Autodesk Fusion 360 part; units mm, degrees
(part 3 of 3)
sketch "Sketch9" plane through (0, 0, 0) normal (1, 0, 0) x (0, 1, 0)
  line L0 (143.1111, 10) -> (156, 10)
  line L1 (156, 10) -> (156, 27)
  line L2 (156, 27) -> (161, 27)
  line L3 (161, 27) -> (161, 49)
  line L4 (161, 49) -> (156, 49)
  line L5 (156, 49) -> (156, 71)
  line L6 (156, 71) -> (161, 71)
  line L7 (161, 71) -> (161, 93)
  line L8 (161, 93) -> (156, 93)
  line L9 (156, 93) -> (156, 115)
  line L10 (156, 115) -> (5, 115)
  line L11 (5, 115) -> (5, 93)
  line L12 (5, 93) -> (0, 93)
  line L13 (0, 93) -> (0, 71)
  line L14 (0, 71) -> (5, 71)
  line L15 (5, 71) -> (5, 49)
  line L16 (5, 49) -> (0, 49)
  line L17 (0, 49) -> (0, 27)
  line L18 (0, 27) -> (5, 27)
  line L19 (5, 27) -> (5, 10)
  line L20 (5, 10) -> (17.8889, 10)
  line L21 (17.8889, 10) -> (17.8889, 5)
  line L22 (17.8889, 5) -> (35.7778, 5)
  line L23 (35.7778, 5) -> (35.7778, 10)
  line L24 (35.7778, 10) -> (53.6667, 10)
  line L25 (53.6667, 10) -> (53.6667, 5)
  line L26 (53.6667, 5) -> (71.5556, 5)
  line L27 (71.5556, 5) -> (71.5556, 10)
  line L28 (71.5556, 10) -> (89.4444, 10)
  line L29 (89.4444, 10) -> (89.4444, 5)
  line L30 (89.4444, 5) -> (107.3333, 5)
  line L31 (107.3333, 5) -> (107.3333, 10)
  line L32 (107.3333, 10) -> (125.2222, 10)
  line L33 (125.2222, 10) -> (125.2222, 5)
  line L34 (125.2222, 5) -> (143.1111, 5)
  line L35 (143.1111, 5) -> (143.1111, 10)
  line L36 (47.6667, 26.5) -> (47.6667, 32.5)
  line L37 (47.6667, 32.5) -> (53.6667, 32.5)
  line L38 (53.6667, 32.5) -> (53.6667, 26.5)
  line L39 (53.6667, 26.5) -> (47.6667, 26.5)
  line L40 (55.3333, 26.5) -> (55.3333, 32.5)
  line L41 (55.3333, 32.5) -> (61.3333, 32.5)
  line L42 (61.3333, 32.5) -> (61.3333, 26.5)
  line L43 (61.3333, 26.5) -> (55.3333, 26.5)
  line L44 (63, 26.5) -> (63, 32.5)
  line L45 (63, 32.5) -> (69, 32.5)
  line L46 (69, 32.5) -> (69, 26.5)
  line L47 (69, 26.5) -> (63, 26.5)
  line L48 (70.6667, 26.5) -> (70.6667, 32.5)
  line L49 (70.6667, 32.5) -> (76.6667, 32.5)
  line L50 (76.6667, 32.5) -> (76.6667, 26.5)
  line L51 (76.6667, 26.5) -> (70.6667, 26.5)
  line L52 (78.3333, 26.5) -> (78.3333, 32.5)
  line L53 (78.3333, 32.5) -> (84.3333, 32.5)
  line L54 (84.3333, 32.5) -> (84.3333, 26.5)
  line L55 (84.3333, 26.5) -> (78.3333, 26.5)
  line L56 (86, 26.5) -> (86, 32.5)
  line L57 (86, 32.5) -> (92, 32.5)
  line L58 (92, 32.5) -> (92, 26.5)
  line L59 (92, 26.5) -> (86, 26.5)
  line L60 (93.6667, 26.5) -> (93.6667, 32.5)
  line L61 (93.6667, 32.5) -> (99.6667, 32.5)
  line L62 (99.6667, 32.5) -> (99.6667, 26.5)
  line L63 (99.6667, 26.5) -> (93.6667, 26.5)
  line L64 (101.3333, 26.5) -> (101.3333, 32.5)
  line L65 (101.3333, 32.5) -> (107.3333, 32.5)
  line L66 (107.3333, 32.5) -> (107.3333, 26.5)
  line L67 (107.3333, 26.5) -> (101.3333, 26.5)
  line L68 (47.6667, 34.3571) -> (47.6667, 40.3571)
  line L69 (47.6667, 40.3571) -> (53.6667, 40.3571)
  line L70 (53.6667, 40.3571) -> (53.6667, 34.3571)
  line L71 (53.6667, 34.3571) -> (47.6667, 34.3571)
  line L72 (55.3333, 34.3571) -> (55.3333, 40.3571)
  line L73 (55.3333, 40.3571) -> (61.3333, 40.3571)
  line L74 (61.3333, 40.3571) -> (61.3333, 34.3571)
  line L75 (61.3333, 34.3571) -> (55.3333, 34.3571)
  line L76 (63, 34.3571) -> (63, 40.3571)
  line L77 (63, 40.3571) -> (69, 40.3571)
  line L78 (69, 40.3571) -> (69, 34.3571)
  line L79 (69, 34.3571) -> (63, 34.3571)
  line L80 (70.6667, 34.3571) -> (70.6667, 40.3571)
  line L81 (70.6667, 40.3571) -> (76.6667, 40.3571)
  line L82 (76.6667, 40.3571) -> (76.6667, 34.3571)
  line L83 (76.6667, 34.3571) -> (70.6667, 34.3571)
  line L84 (78.3333, 34.3571) -> (78.3333, 40.3571)
  line L85 (78.3333, 40.3571) -> (84.3333, 40.3571)
  line L86 (84.3333, 40.3571) -> (84.3333, 34.3571)
  line L87 (84.3333, 34.3571) -> (78.3333, 34.3571)
  line L88 (86, 34.3571) -> (86, 40.3571)
  line L89 (86, 40.3571) -> (92, 40.3571)
  line L90 (92, 40.3571) -> (92, 34.3571)
  line L91 (92, 34.3571) -> (86, 34.3571)
  line L92 (93.6667, 34.3571) -> (93.6667, 40.3571)
  line L93 (93.6667, 40.3571) -> (99.6667, 40.3571)
  line L94 (99.6667, 40.3571) -> (99.6667, 34.3571)
  line L95 (99.6667, 34.3571) -> (93.6667, 34.3571)
  line L96 (101.3333, 34.3571) -> (101.3333, 40.3571)
  line L97 (101.3333, 40.3571) -> (107.3333, 40.3571)
  line L98 (107.3333, 40.3571) -> (107.3333, 34.3571)
  line L99 (107.3333, 34.3571) -> (101.3333, 34.3571)
  line L100 (47.6667, 42.2143) -> (47.6667, 48.2143)
  line L101 (47.6667, 48.2143) -> (53.6667, 48.2143)
  line L102 (53.6667, 48.2143) -> (53.6667, 42.2143)
  line L103 (53.6667, 42.2143) -> (47.6667, 42.2143)
  line L104 (55.3333, 42.2143) -> (55.3333, 48.2143)
  line L105 (55.3333, 48.2143) -> (61.3333, 48.2143)
  line L106 (61.3333, 48.2143) -> (61.3333, 42.2143)
  line L107 (61.3333, 42.2143) -> (55.3333, 42.2143)
  line L108 (63, 42.2143) -> (63, 48.2143)
  line L109 (63, 48.2143) -> (69, 48.2143)
  line L110 (69, 48.2143) -> (69, 42.2143)
  line L111 (69, 42.2143) -> (63, 42.2143)
  line L112 (70.6667, 42.2143) -> (70.6667, 48.2143)
  line L113 (70.6667, 48.2143) -> (76.6667, 48.2143)
  line L114 (76.6667, 48.2143) -> (76.6667, 42.2143)
  line L115 (76.6667, 42.2143) -> (70.6667, 42.2143)
  line L116 (78.3333, 42.2143) -> (78.3333, 48.2143)
  line L117 (78.3333, 48.2143) -> (84.3333, 48.2143)
  line L118 (84.3333, 48.2143) -> (84.3333, 42.2143)
  line L119 (84.3333, 42.2143) -> (78.3333, 42.2143)
  line L120 (86, 42.2143) -> (86, 48.2143)
  line L121 (86, 48.2143) -> (92, 48.2143)
  line L122 (92, 48.2143) -> (92, 42.2143)
  line L123 (92, 42.2143) -> (86, 42.2143)
  line L124 (93.6667, 42.2143) -> (93.6667, 48.2143)
  line L125 (93.6667, 48.2143) -> (99.6667, 48.2143)
  line L126 (99.6667, 48.2143) -> (99.6667, 42.2143)
  line L127 (99.6667, 42.2143) -> (93.6667, 42.2143)
  line L128 (101.3333, 42.2143) -> (101.3333, 48.2143)
  line L129 (101.3333, 48.2143) -> (107.3333, 48.2143)
  line L130 (107.3333, 48.2143) -> (107.3333, 42.2143)
  line L131 (107.3333, 42.2143) -> (101.3333, 42.2143)
  line L132 (47.6667, 50.0714) -> (47.6667, 56.0714)
  line L133 (47.6667, 56.0714) -> (53.6667, 56.0714)
  line L134 (53.6667, 56.0714) -> (53.6667, 50.0714)
  line L135 (53.6667, 50.0714) -> (47.6667, 50.0714)
  line L136 (55.3333, 50.0714) -> (55.3333, 56.0714)
  line L137 (55.3333, 56.0714) -> (61.3333, 56.0714)
  line L138 (61.3333, 56.0714) -> (61.3333, 50.0714)
  line L139 (61.3333, 50.0714) -> (55.3333, 50.0714)
  line L140 (63, 50.0714) -> (63, 56.0714)
  line L141 (63, 56.0714) -> (69, 56.0714)
  line L142 (69, 56.0714) -> (69, 50.0714)
  line L143 (69, 50.0714) -> (63, 50.0714)
  line L144 (70.6667, 50.0714) -> (70.6667, 56.0714)
  line L145 (70.6667, 56.0714) -> (76.6667, 56.0714)
  line L146 (76.6667, 56.0714) -> (76.6667, 50.0714)
  line L147 (76.6667, 50.0714) -> (70.6667, 50.0714)
  line L148 (78.3333, 50.0714) -> (78.3333, 56.0714)
  line L149 (78.3333, 56.0714) -> (84.3333, 56.0714)
  line L150 (84.3333, 56.0714) -> (84.3333, 50.0714)
  line L151 (84.3333, 50.0714) -> (78.3333, 50.0714)
  line L152 (86, 50.0714) -> (86, 56.0714)
  line L153 (86, 56.0714) -> (92, 56.0714)
  line L154 (92, 56.0714) -> (92, 50.0714)
  line L155 (92, 50.0714) -> (86, 50.0714)
  line L156 (93.6667, 50.0714) -> (93.6667, 56.0714)
  line L157 (93.6667, 56.0714) -> (99.6667, 56.0714)
  line L158 (99.6667, 56.0714) -> (99.6667, 50.0714)
  line L159 (99.6667, 50.0714) -> (93.6667, 50.0714)
  line L160 (101.3333, 50.0714) -> (101.3333, 56.0714)
  line L161 (101.3333, 56.0714) -> (107.3333, 56.0714)
  line L162 (107.3333, 56.0714) -> (107.3333, 50.0714)
  line L163 (107.3333, 50.0714) -> (101.3333, 50.0714)
  line L164 (47.6667, 57.9286) -> (47.6667, 63.9286)
  line L165 (47.6667, 63.9286) -> (53.6667, 63.9286)
  line L166 (53.6667, 63.9286) -> (53.6667, 57.9286)
  line L167 (53.6667, 57.9286) -> (47.6667, 57.9286)
  line L168 (55.3333, 57.9286) -> (55.3333, 63.9286)
  line L169 (55.3333, 63.9286) -> (61.3333, 63.9286)
  line L170 (61.3333, 63.9286) -> (61.3333, 57.9286)
  line L171 (61.3333, 57.9286) -> (55.3333, 57.9286)
  line L172 (63, 57.9286) -> (63, 63.9286)
  line L173 (63, 63.9286) -> (69, 63.9286)
  line L174 (69, 63.9286) -> (69, 57.9286)
  line L175 (69, 57.9286) -> (63, 57.9286)
  line L176 (70.6667, 57.9286) -> (70.6667, 63.9286)
  line L177 (70.6667, 63.9286) -> (76.6667, 63.9286)
  line L178 (76.6667, 63.9286) -> (76.6667, 57.9286)
  line L179 (76.6667, 57.9286) -> (70.6667, 57.9286)
  line L180 (78.3333, 57.9286) -> (78.3333, 63.9286)
  line L181 (78.3333, 63.9286) -> (84.3333, 63.9286)
  line L182 (84.3333, 63.9286) -> (84.3333, 57.9286)
  line L183 (84.3333, 57.9286) -> (78.3333, 57.9286)
  line L184 (86, 57.9286) -> (86, 63.9286)
  line L185 (86, 63.9286) -> (92, 63.9286)
  line L186 (92, 63.9286) -> (92, 57.9286)
  line L187 (92, 57.9286) -> (86, 57.9286)
  line L188 (93.6667, 57.9286) -> (93.6667, 63.9286)
  line L189 (93.6667, 63.9286) -> (99.6667, 63.9286)
  line L190 (99.6667, 63.9286) -> (99.6667, 57.9286)
  line L191 (99.6667, 57.9286) -> (93.6667, 57.9286)
  line L192 (101.3333, 57.9286) -> (101.3333, 63.9286)
  line L193 (101.3333, 63.9286) -> (107.3333, 63.9286)
  line L194 (107.3333, 63.9286) -> (107.3333, 57.9286)
  line L195 (107.3333, 57.9286) -> (101.3333, 57.9286)
  line L196 (47.6667, 65.7857) -> (47.6667, 71.7857)
  line L197 (47.6667, 71.7857) -> (53.6667, 71.7857)
  line L198 (53.6667, 71.7857) -> (53.6667, 65.7857)
  line L199 (53.6667, 65.7857) -> (47.6667, 65.7857)
  line L200 (55.3333, 65.7857) -> (55.3333, 71.7857)
  line L201 (55.3333, 71.7857) -> (61.3333, 71.7857)
  line L202 (61.3333, 71.7857) -> (61.3333, 65.7857)
  line L203 (61.3333, 65.7857) -> (55.3333, 65.7857)
  line L204 (63, 65.7857) -> (63, 71.7857)
  line L205 (63, 71.7857) -> (69, 71.7857)
  line L206 (69, 71.7857) -> (69, 65.7857)
  line L207 (69, 65.7857) -> (63, 65.7857)
  line L208 (70.6667, 65.7857) -> (70.6667, 71.7857)
  line L209 (70.6667, 71.7857) -> (76.6667, 71.7857)
  line L210 (76.6667, 71.7857) -> (76.6667, 65.7857)
  line L211 (76.6667, 65.7857) -> (70.6667, 65.7857)
  line L212 (78.3333, 65.7857) -> (78.3333, 71.7857)
  line L213 (78.3333, 71.7857) -> (84.3333, 71.7857)
  line L214 (84.3333, 71.7857) -> (84.3333, 65.7857)
  line L215 (84.3333, 65.7857) -> (78.3333, 65.7857)
  line L216 (86, 65.7857) -> (86, 71.7857)
  line L217 (86, 71.7857) -> (92, 71.7857)
  line L218 (92, 71.7857) -> (92, 65.7857)
  line L219 (92, 65.7857) -> (86, 65.7857)
  line L220 (93.6667, 65.7857) -> (93.6667, 71.7857)
  line L221 (93.6667, 71.7857) -> (99.6667, 71.7857)
  line L222 (99.6667, 71.7857) -> (99.6667, 65.7857)
  line L223 (99.6667, 65.7857) -> (93.6667, 65.7857)
  line L224 (101.3333, 65.7857) -> (101.3333, 71.7857)
  line L225 (101.3333, 71.7857) -> (107.3333, 71.7857)
  line L226 (107.3333, 71.7857) -> (107.3333, 65.7857)
  line L227 (107.3333, 65.7857) -> (101.3333, 65.7857)
  line L228 (47.6667, 73.6429) -> (47.6667, 79.6429)
  line L229 (47.6667, 79.6429) -> (53.6667, 79.6429)
  line L230 (53.6667, 79.6429) -> (53.6667, 73.6429)
  line L231 (53.6667, 73.6429) -> (47.6667, 73.6429)
  line L232 (55.3333, 73.6429) -> (55.3333, 79.6429)
  line L233 (55.3333, 79.6429) -> (61.3333, 79.6429)
  line L234 (61.3333, 79.6429) -> (61.3333, 73.6429)
  line L235 (61.3333, 73.6429) -> (55.3333, 73.6429)
  line L236 (63, 73.6429) -> (63, 79.6429)
  line L237 (63, 79.6429) -> (69, 79.6429)
  line L238 (69, 79.6429) -> (69, 73.6429)
  line L239 (69, 73.6429) -> (63, 73.6429)
  line L240 (70.6667, 73.6429) -> (70.6667, 79.6429)
  line L241 (70.6667, 79.6429) -> (76.6667, 79.6429)
  line L242 (76.6667, 79.6429) -> (76.6667, 73.6429)
  line L243 (76.6667, 73.6429) -> (70.6667, 73.6429)
  line L244 (78.3333, 73.6429) -> (78.3333, 79.6429)
  line L245 (78.3333, 79.6429) -> (84.3333, 79.6429)
  line L246 (84.3333, 79.6429) -> (84.3333, 73.6429)
  line L247 (84.3333, 73.6429) -> (78.3333, 73.6429)
  line L248 (86, 73.6429) -> (86, 79.6429)
  line L249 (86, 79.6429) -> (92, 79.6429)
  line L250 (92, 79.6429) -> (92, 73.6429)
  line L251 (92, 73.6429) -> (86, 73.6429)
  line L252 (93.6667, 73.6429) -> (93.6667, 79.6429)
  line L253 (93.6667, 79.6429) -> (99.6667, 79.6429)
  line L254 (99.6667, 79.6429) -> (99.6667, 73.6429)
  line L255 (99.6667, 73.6429) -> (93.6667, 73.6429)
  line L256 (101.3333, 73.6429) -> (101.3333, 79.6429)
  line L257 (101.3333, 79.6429) -> (107.3333, 79.6429)
  line L258 (107.3333, 79.6429) -> (107.3333, 73.6429)
  line L259 (107.3333, 73.6429) -> (101.3333, 73.6429)
  line L260 (47.6667, 81.5) -> (47.6667, 87.5)
  line L261 (47.6667, 87.5) -> (53.6667, 87.5)
  line L262 (53.6667, 87.5) -> (53.6667, 81.5)
  line L263 (53.6667, 81.5) -> (47.6667, 81.5)
  line L264 (55.3333, 81.5) -> (55.3333, 87.5)
  line L265 (55.3333, 87.5) -> (61.3333, 87.5)
  line L266 (61.3333, 87.5) -> (61.3333, 81.5)
  line L267 (61.3333, 81.5) -> (55.3333, 81.5)
  line L268 (63, 81.5) -> (63, 87.5)
  line L269 (63, 87.5) -> (69, 87.5)
  line L270 (69, 87.5) -> (69, 81.5)
  line L271 (69, 81.5) -> (63, 81.5)
  line L272 (70.6667, 81.5) -> (70.6667, 87.5)
  line L273 (70.6667, 87.5) -> (76.6667, 87.5)
  line L274 (76.6667, 87.5) -> (76.6667, 81.5)
  line L275 (76.6667, 81.5) -> (70.6667, 81.5)
  line L276 (78.3333, 81.5) -> (78.3333, 87.5)
  line L277 (78.3333, 87.5) -> (84.3333, 87.5)
  line L278 (84.3333, 87.5) -> (84.3333, 81.5)
  line L279 (84.3333, 81.5) -> (78.3333, 81.5)
  line L280 (86, 81.5) -> (86, 87.5)
  line L281 (86, 87.5) -> (92, 87.5)
  line L282 (92, 87.5) -> (92, 81.5)
  line L283 (92, 81.5) -> (86, 81.5)
  line L284 (93.6667, 81.5) -> (93.6667, 87.5)
  line L285 (93.6667, 87.5) -> (99.6667, 87.5)
  line L286 (99.6667, 87.5) -> (99.6667, 81.5)
  line L287 (99.6667, 81.5) -> (93.6667, 81.5)
  line L288 (107.3333, 87.5) -> (107.3333, 81.5)
  line L289 (107.3333, 81.5) -> (101.3333, 81.5)
  line L290 (101.3333, 81.5) -> (101.3333, 87.5)
  line L291 (101.3333, 87.5) -> (107.3333, 87.5)
  line L292 (199.3333, -50) -> (184.3333, -50)
  line L293 (184.3333, -50) -> (184.3333, -44)
  line L294 (184.3333, -44) -> (199.3333, -44)
  line L295 (199.3333, -44) -> (199.3333, -50)
  line L296 (199.3333, -58.3333) -> (184.3333, -58.3333)
  line L297 (184.3333, -58.3333) -> (184.3333, -52.3333)
  line L298 (184.3333, -52.3333) -> (199.3333, -52.3333)
  line L299 (199.3333, -52.3333) -> (199.3333, -58.3333)
  line L300 (199.3333, -66.6667) -> (184.3333, -66.6667)
  line L301 (184.3333, -66.6667) -> (184.3333, -60.6667)
  line L302 (184.3333, -60.6667) -> (199.3333, -60.6667)
  line L303 (199.3333, -60.6667) -> (199.3333, -66.6667)
  line L304 (199.3333, -75) -> (184.3333, -75)
  line L305 (184.3333, -75) -> (184.3333, -69)
  line L306 (184.3333, -69) -> (199.3333, -69)
  line L307 (199.3333, -69) -> (199.3333, -75)
  line L308 (199.3333, -83.3333) -> (184.3333, -83.3333)
  line L309 (184.3333, -83.3333) -> (184.3333, -77.3333)
  line L310 (184.3333, -77.3333) -> (199.3333, -77.3333)
  line L311 (199.3333, -77.3333) -> (199.3333, -83.3333)
  line L312 (199.3333, -91.6667) -> (184.3333, -91.6667)
  line L313 (184.3333, -91.6667) -> (184.3333, -85.6667)
  line L314 (184.3333, -85.6667) -> (199.3333, -85.6667)
  line L315 (199.3333, -85.6667) -> (199.3333, -91.6667)
  line L316 (199.3333, -100) -> (184.3333, -100)
  line L317 (184.3333, -100) -> (184.3333, -94)
  line L318 (184.3333, -94) -> (199.3333, -94)
  line L319 (199.3333, -94) -> (199.3333, -100)
  line L320 (199.3333, -108.3333) -> (184.3333, -108.3333)
  line L321 (184.3333, -108.3333) -> (184.3333, -102.3333)
  line L322 (184.3333, -102.3333) -> (199.3333, -102.3333)
  line L323 (199.3333, -102.3333) -> (199.3333, -108.3333)
  line L324 (199.3333, -116.6667) -> (184.3333, -116.6667)
  line L325 (184.3333, -116.6667) -> (184.3333, -110.6667)
  line L326 (184.3333, -110.6667) -> (199.3333, -110.6667)
  line L327 (199.3333, -110.6667) -> (199.3333, -116.6667)
  line L328 (199.3333, -125) -> (184.3333, -125)
  line L329 (184.3333, -125) -> (184.3333, -119)
  line L330 (184.3333, -119) -> (199.3333, -119)
  line L331 (199.3333, -119) -> (199.3333, -125)
  line L332 (188, -5) -> (188, 0)
  line L333 (188, 0) -> (171, 0)
  line L334 (171, 0) -> (171, -13.6364)
  line L335 (171, -13.6364) -> (166, -13.6364)
  line L336 (166, -13.6364) -> (166, -27.2727)
  line L337 (166, -27.2727) -> (171, -27.2727)
  line L338 (171, -27.2727) -> (171, -40.9091)
  line L339 (171, -40.9091) -> (166, -40.9091)
  line L340 (166, -40.9091) -> (166, -54.5455)
  line L341 (166, -54.5455) -> (171, -54.5455)
  line L342 (171, -54.5455) -> (171, -68.1818)
  line L343 (171, -68.1818) -> (166, -68.1818)
  line L344 (166, -68.1818) -> (166, -81.8182)
  line L345 (166, -81.8182) -> (171, -81.8182)
  line L346 (171, -81.8182) -> (171, -95.4545)
  line L347 (171, -95.4545) -> (166, -95.4545)
  line L348 (166, -95.4545) -> (166, -109.0909)
  line L349 (166, -109.0909) -> (171, -109.0909)
  line L350 (171, -109.0909) -> (171, -122.7273)
  line L351 (171, -122.7273) -> (166, -122.7273)
  line L352 (166, -122.7273) -> (166, -136.3636)
  line L353 (166, -136.3636) -> (171, -136.3636)
  line L354 (171, -136.3636) -> (171, -150)
  line L355 (171, -150) -> (188, -150)
  line L356 (188, -150) -> (188, -145)
  line L357 (188, -145) -> (210, -145)
  line L358 (210, -145) -> (210, -150)
  line L359 (210, -150) -> (232, -150)
  line L360 (232, -150) -> (232, -145)
  line L361 (232, -145) -> (254, -145)
  line L362 (254, -145) -> (254, -150)
  line L363 (254, -150) -> (276, -150)
  line L364 (276, -150) -> (276, 0)
  line L365 (276, 0) -> (254, 0)
  line L366 (254, 0) -> (254, -5)
  line L367 (254, -5) -> (232, -5)
  line L368 (232, -5) -> (232, 0)
  line L369 (232, 0) -> (210, 0)
  line L370 (210, 0) -> (210, -5)
  line L371 (210, -5) -> (188, -5)
  line L372 (17.8889, -5) -> (17.8889, 0)
  line L373 (17.8889, 0) -> (0, 0)
  line L374 (0, 0) -> (0, -13.6364)
  line L375 (0, -13.6364) -> (5, -13.6364)
  line L376 (5, -13.6364) -> (5, -27.2727)
  line L377 (5, -27.2727) -> (0, -27.2727)
  line L378 (0, -27.2727) -> (0, -40.9091)
  line L379 (0, -40.9091) -> (5, -40.9091)
  line L380 (5, -40.9091) -> (5, -54.5455)
  line L381 (5, -54.5455) -> (0, -54.5455)
  line L382 (0, -54.5455) -> (0, -68.1818)
  line L383 (0, -68.1818) -> (5, -68.1818)
  line L384 (5, -68.1818) -> (5, -81.8182)
  line L385 (5, -81.8182) -> (0, -81.8182)
  line L386 (0, -81.8182) -> (0, -95.4545)
  line L387 (0, -95.4545) -> (5, -95.4545)
  line L388 (5, -95.4545) -> (5, -109.0909)
  line L389 (5, -109.0909) -> (0, -109.0909)
  line L390 (0, -109.0909) -> (0, -122.7273)
  line L391 (0, -122.7273) -> (5, -122.7273)
  line L392 (5, -122.7273) -> (5, -136.3636)
  line L393 (5, -136.3636) -> (0, -136.3636)
  line L394 (0, -136.3636) -> (0, -150)
  line L395 (0, -150) -> (17.8889, -150)
  line L396 (17.8889, -150) -> (17.8889, -145)
  line L397 (17.8889, -145) -> (35.7778, -145)
  line L398 (35.7778, -145) -> (35.7778, -150)
  line L399 (35.7778, -150) -> (53.6667, -150)
  line L400 (53.6667, -150) -> (53.6667, -145)
  line L401 (53.6667, -145) -> (71.5556, -145)
  line L402 (71.5556, -145) -> (71.5556, -150)
  line L403 (71.5556, -150) -> (89.4444, -150)
  line L404 (89.4444, -150) -> (89.4444, -145)
  line L405 (89.4444, -145) -> (107.3333, -145)
  line L406 (107.3333, -145) -> (107.3333, -150)
  line L407 (107.3333, -150) -> (125.2222, -150)
  line L408 (125.2222, -150) -> (125.2222, -145)
  line L409 (125.2222, -145) -> (143.1111, -145)
  line L410 (143.1111, -145) -> (143.1111, -150)
  line L411 (143.1111, -150) -> (161, -150)
  line L412 (161, -150) -> (161, -136.3636)
  line L413 (161, -136.3636) -> (156, -136.3636)
  line L414 (156, -136.3636) -> (156, -122.7273)
  line L415 (156, -122.7273) -> (161, -122.7273)
  line L416 (161, -122.7273) -> (161, -109.0909)
  line L417 (161, -109.0909) -> (156, -109.0909)
  line L418 (156, -109.0909) -> (156, -95.4545)
  line L419 (156, -95.4545) -> (161, -95.4545)
  line L420 (161, -95.4545) -> (161, -81.8182)
  line L421 (161, -81.8182) -> (156, -81.8182)
  line L422 (156, -81.8182) -> (156, -68.1818)
  line L423 (156, -68.1818) -> (161, -68.1818)
  line L424 (161, -68.1818) -> (161, -54.5455)
  line L425 (161, -54.5455) -> (156, -54.5455)
  line L426 (156, -54.5455) -> (156, -40.9091)
  line L427 (156, -40.9091) -> (161, -40.9091)
  line L428 (161, -40.9091) -> (161, -27.2727)
  line L429 (161, -27.2727) -> (156, -27.2727)
  line L430 (156, -27.2727) -> (156, -13.6364)
  line L431 (156, -13.6364) -> (161, -13.6364)
  line L432 (161, -13.6364) -> (161, 0)
  line L433 (161, 0) -> (143.1111, 0)
  line L434 (143.1111, 0) -> (143.1111, -5)
  line L435 (143.1111, -5) -> (125.2222, -5)
  line L436 (125.2222, -5) -> (125.2222, 0)
  line L437 (125.2222, 0) -> (107.3333, 0)
  line L438 (107.3333, 0) -> (107.3333, -5)
  line L439 (107.3333, -5) -> (89.4444, -5)
  line L440 (89.4444, -5) -> (89.4444, 0)
  line L441 (89.4444, 0) -> (71.5556, 0)
  line L442 (71.5556, 0) -> (71.5556, -5)
  line L443 (71.5556, -5) -> (53.6667, -5)
  line L444 (53.6667, -5) -> (53.6667, 0)
  line L445 (53.6667, 0) -> (35.7778, 0)
  line L446 (35.7778, 0) -> (35.7778, -5)
  line L447 (35.7778, -5) -> (17.8889, -5)
  line L448 (53.6667, -182.5) -> (47.6667, -182.5)
  line L449 (47.6667, -182.5) -> (47.6667, -176.5)
  line L450 (47.6667, -176.5) -> (53.6667, -176.5)
  line L451 (53.6667, -176.5) -> (53.6667, -182.5)
  line L452 (61.3333, -182.5) -> (55.3333, -182.5)
  line L453 (55.3333, -182.5) -> (55.3333, -176.5)
  line L454 (55.3333, -176.5) -> (61.3333, -176.5)
  line L455 (61.3333, -176.5) -> (61.3333, -182.5)
  line L456 (69, -182.5) -> (63, -182.5)
  line L457 (63, -182.5) -> (63, -176.5)
  line L458 (63, -176.5) -> (69, -176.5)
  line L459 (69, -176.5) -> (69, -182.5)
  line L460 (76.6667, -182.5) -> (70.6667, -182.5)
  line L461 (70.6667, -182.5) -> (70.6667, -176.5)
  line L462 (70.6667, -176.5) -> (76.6667, -176.5)
  line L463 (76.6667, -176.5) -> (76.6667, -182.5)
  line L464 (84.3333, -182.5) -> (78.3333, -182.5)
  line L465 (78.3333, -182.5) -> (78.3333, -176.5)
  line L466 (78.3333, -176.5) -> (84.3333, -176.5)
  line L467 (84.3333, -176.5) -> (84.3333, -182.5)
  line L468 (92, -182.5) -> (86, -182.5)
  line L469 (86, -182.5) -> (86, -176.5)
  line L470 (86, -176.5) -> (92, -176.5)
  line L471 (92, -176.5) -> (92, -182.5)
  line L472 (99.6667, -182.5) -> (93.6667, -182.5)
  line L473 (93.6667, -182.5) -> (93.6667, -176.5)
  line L474 (93.6667, -176.5) -> (99.6667, -176.5)
  line L475 (99.6667, -176.5) -> (99.6667, -182.5)
  line L476 (107.3333, -182.5) -> (101.3333, -182.5)
  line L477 (101.3333, -182.5) -> (101.3333, -176.5)
  line L478 (101.3333, -176.5) -> (107.3333, -176.5)
  line L479 (107.3333, -176.5) -> (107.3333, -182.5)
  line L480 (53.6667, -190.3571) -> (47.6667, -190.3571)
  line L481 (47.6667, -190.3571) -> (47.6667, -184.3571)
  line L482 (47.6667, -184.3571) -> (53.6667, -184.3571)
  line L483 (53.6667, -184.3571) -> (53.6667, -190.3571)
  line L484 (61.3333, -190.3571) -> (55.3333, -190.3571)
  line L485 (55.3333, -190.3571) -> (55.3333, -184.3571)
  line L486 (55.3333, -184.3571) -> (61.3333, -184.3571)
  line L487 (61.3333, -184.3571) -> (61.3333, -190.3571)
  line L488 (69, -190.3571) -> (63, -190.3571)
  line L489 (63, -190.3571) -> (63, -184.3571)
  line L490 (63, -184.3571) -> (69, -184.3571)
  line L491 (69, -184.3571) -> (69, -190.3571)
  line L492 (76.6667, -190.3571) -> (70.6667, -190.3571)
  line L493 (70.6667, -190.3571) -> (70.6667, -184.3571)
  line L494 (70.6667, -184.3571) -> (76.6667, -184.3571)
  line L495 (76.6667, -184.3571) -> (76.6667, -190.3571)
  line L496 (84.3333, -190.3571) -> (78.3333, -190.3571)
  line L497 (78.3333, -190.3571) -> (78.3333, -184.3571)
  line L498 (78.3333, -184.3571) -> (84.3333, -184.3571)
  line L499 (84.3333, -184.3571) -> (84.3333, -190.3571)
  line L500 (92, -190.3571) -> (86, -190.3571)
  line L501 (86, -190.3571) -> (86, -184.3571)
  line L502 (86, -184.3571) -> (92, -184.3571)
  line L503 (92, -184.3571) -> (92, -190.3571)
  line L504 (99.6667, -190.3571) -> (93.6667, -190.3571)
  line L505 (93.6667, -190.3571) -> (93.6667, -184.3571)
  line L506 (93.6667, -184.3571) -> (99.6667, -184.3571)
  line L507 (99.6667, -184.3571) -> (99.6667, -190.3571)
  line L508 (107.3333, -190.3571) -> (101.3333, -190.3571)
  line L509 (101.3333, -190.3571) -> (101.3333, -184.3571)
  line L510 (101.3333, -184.3571) -> (107.3333, -184.3571)
  line L511 (107.3333, -184.3571) -> (107.3333, -190.3571)
  line L512 (53.6667, -198.2143) -> (47.6667, -198.2143)
  line L513 (47.6667, -198.2143) -> (47.6667, -192.2143)
  line L514 (47.6667, -192.2143) -> (53.6667, -192.2143)
  line L515 (53.6667, -192.2143) -> (53.6667, -198.2143)
  line L516 (61.3333, -198.2143) -> (55.3333, -198.2143)
  line L517 (55.3333, -198.2143) -> (55.3333, -192.2143)
  line L518 (55.3333, -192.2143) -> (61.3333, -192.2143)
  line L519 (61.3333, -192.2143) -> (61.3333, -198.2143)
  line L520 (69, -198.2143) -> (63, -198.2143)
  line L521 (63, -198.2143) -> (63, -192.2143)
  line L522 (63, -192.2143) -> (69, -192.2143)
  line L523 (69, -192.2143) -> (69, -198.2143)
  line L524 (76.6667, -198.2143) -> (70.6667, -198.2143)
  line L525 (70.6667, -198.2143) -> (70.6667, -192.2143)
  line L526 (70.6667, -192.2143) -> (76.6667, -192.2143)
  line L527 (76.6667, -192.2143) -> (76.6667, -198.2143)
  line L528 (84.3333, -198.2143) -> (78.3333, -198.2143)
  line L529 (78.3333, -198.2143) -> (78.3333, -192.2143)
  line L530 (78.3333, -192.2143) -> (84.3333, -192.2143)
  line L531 (84.3333, -192.2143) -> (84.3333, -198.2143)
  line L532 (92, -198.2143) -> (86, -198.2143)
  line L533 (86, -198.2143) -> (86, -192.2143)
  line L534 (86, -192.2143) -> (92, -192.2143)
  line L535 (92, -192.2143) -> (92, -198.2143)
  line L536 (99.6667, -198.2143) -> (93.6667, -198.2143)
  line L537 (93.6667, -198.2143) -> (93.6667, -192.2143)
  line L538 (93.6667, -192.2143) -> (99.6667, -192.2143)
  line L539 (99.6667, -192.2143) -> (99.6667, -198.2143)
  line L540 (107.3333, -198.2143) -> (101.3333, -198.2143)
  line L541 (101.3333, -198.2143) -> (101.3333, -192.2143)
  line L542 (101.3333, -192.2143) -> (107.3333, -192.2143)
  line L543 (107.3333, -192.2143) -> (107.3333, -198.2143)
  line L544 (53.6667, -206.0714) -> (47.6667, -206.0714)
  line L545 (47.6667, -206.0714) -> (47.6667, -200.0714)
  line L546 (47.6667, -200.0714) -> (53.6667, -200.0714)
  line L547 (53.6667, -200.0714) -> (53.6667, -206.0714)
  line L548 (61.3333, -206.0714) -> (55.3333, -206.0714)
  line L549 (55.3333, -206.0714) -> (55.3333, -200.0714)
  line L550 (55.3333, -200.0714) -> (61.3333, -200.0714)
  line L551 (61.3333, -200.0714) -> (61.3333, -206.0714)
  line L552 (69, -206.0714) -> (63, -206.0714)
  line L553 (63, -206.0714) -> (63, -200.0714)
  line L554 (63, -200.0714) -> (69, -200.0714)
  line L555 (69, -200.0714) -> (69, -206.0714)
  line L556 (76.6667, -206.0714) -> (70.6667, -206.0714)
  line L557 (70.6667, -206.0714) -> (70.6667, -200.0714)
  line L558 (70.6667, -200.0714) -> (76.6667, -200.0714)
  line L559 (76.6667, -200.0714) -> (76.6667, -206.0714)
  line L560 (84.3333, -206.0714) -> (78.3333, -206.0714)
  line L561 (78.3333, -206.0714) -> (78.3333, -200.0714)
  line L562 (78.3333, -200.0714) -> (84.3333, -200.0714)
  line L563 (84.3333, -200.0714) -> (84.3333, -206.0714)
  line L564 (92, -206.0714) -> (86, -206.0714)
  line L565 (86, -206.0714) -> (86, -200.0714)
  line L566 (86, -200.0714) -> (92, -200.0714)
  line L567 (92, -200.0714) -> (92, -206.0714)
  line L568 (99.6667, -206.0714) -> (93.6667, -206.0714)
  line L569 (93.6667, -206.0714) -> (93.6667, -200.0714)
  line L570 (93.6667, -200.0714) -> (99.6667, -200.0714)
  line L571 (99.6667, -200.0714) -> (99.6667, -206.0714)
  line L572 (107.3333, -206.0714) -> (101.3333, -206.0714)
  line L573 (101.3333, -206.0714) -> (101.3333, -200.0714)
  line L574 (101.3333, -200.0714) -> (107.3333, -200.0714)
  line L575 (107.3333, -200.0714) -> (107.3333, -206.0714)
  line L576 (53.6667, -213.9286) -> (47.6667, -213.9286)
  line L577 (47.6667, -213.9286) -> (47.6667, -207.9286)
  line L578 (47.6667, -207.9286) -> (53.6667, -207.9286)
  line L579 (53.6667, -207.9286) -> (53.6667, -213.9286)
  line L580 (61.3333, -213.9286) -> (55.3333, -213.9286)
  line L581 (55.3333, -213.9286) -> (55.3333, -207.9286)
  line L582 (55.3333, -207.9286) -> (61.3333, -207.9286)
  line L583 (61.3333, -207.9286) -> (61.3333, -213.9286)
  line L584 (69, -213.9286) -> (63, -213.9286)
  line L585 (63, -213.9286) -> (63, -207.9286)
  line L586 (63, -207.9286) -> (69, -207.9286)
  line L587 (69, -207.9286) -> (69, -213.9286)
  line L588 (76.6667, -213.9286) -> (70.6667, -213.9286)
  line L589 (70.6667, -213.9286) -> (70.6667, -207.9286)
  line L590 (70.6667, -207.9286) -> (76.6667, -207.9286)
  line L591 (76.6667, -207.9286) -> (76.6667, -213.9286)
  line L592 (84.3333, -213.9286) -> (78.3333, -213.9286)
  line L593 (78.3333, -213.9286) -> (78.3333, -207.9286)
  line L594 (78.3333, -207.9286) -> (84.3333, -207.9286)
  line L595 (84.3333, -207.9286) -> (84.3333, -213.9286)
  line L596 (92, -213.9286) -> (86, -213.9286)
  line L597 (86, -213.9286) -> (86, -207.9286)
  line L598 (86, -207.9286) -> (92, -207.9286)
  line L599 (92, -207.9286) -> (92, -213.9286)
  line L600 (99.6667, -213.9286) -> (93.6667, -213.9286)
  line L601 (93.6667, -213.9286) -> (93.6667, -207.9286)
  line L602 (93.6667, -207.9286) -> (99.6667, -207.9286)
  line L603 (99.6667, -207.9286) -> (99.6667, -213.9286)
  line L604 (107.3333, -213.9286) -> (101.3333, -213.9286)
  line L605 (101.3333, -213.9286) -> (101.3333, -207.9286)
  line L606 (101.3333, -207.9286) -> (107.3333, -207.9286)
  line L607 (107.3333, -207.9286) -> (107.3333, -213.9286)
  line L608 (53.6667, -221.7857) -> (47.6667, -221.7857)
  line L609 (47.6667, -221.7857) -> (47.6667, -215.7857)
  line L610 (47.6667, -215.7857) -> (53.6667, -215.7857)
  line L611 (53.6667, -215.7857) -> (53.6667, -221.7857)
  line L612 (61.3333, -221.7857) -> (55.3333, -221.7857)
  line L613 (55.3333, -221.7857) -> (55.3333, -215.7857)
  line L614 (55.3333, -215.7857) -> (61.3333, -215.7857)
  line L615 (61.3333, -215.7857) -> (61.3333, -221.7857)
  line L616 (69, -221.7857) -> (63, -221.7857)
  line L617 (63, -221.7857) -> (63, -215.7857)
  line L618 (63, -215.7857) -> (69, -215.7857)
  line L619 (69, -215.7857) -> (69, -221.7857)
  line L620 (76.6667, -221.7857) -> (70.6667, -221.7857)
  line L621 (70.6667, -221.7857) -> (70.6667, -215.7857)
  line L622 (70.6667, -215.7857) -> (76.6667, -215.7857)
  line L623 (76.6667, -215.7857) -> (76.6667, -221.7857)
  line L624 (84.3333, -221.7857) -> (78.3333, -221.7857)
  line L625 (78.3333, -221.7857) -> (78.3333, -215.7857)
  line L626 (78.3333, -215.7857) -> (84.3333, -215.7857)
  line L627 (84.3333, -215.7857) -> (84.3333, -221.7857)
  line L628 (92, -221.7857) -> (86, -221.7857)
  line L629 (86, -221.7857) -> (86, -215.7857)
  line L630 (86, -215.7857) -> (92, -215.7857)
  line L631 (92, -215.7857) -> (92, -221.7857)
  line L632 (99.6667, -221.7857) -> (93.6667, -221.7857)
  line L633 (93.6667, -221.7857) -> (93.6667, -215.7857)
  line L634 (93.6667, -215.7857) -> (99.6667, -215.7857)
  line L635 (99.6667, -215.7857) -> (99.6667, -221.7857)
  line L636 (107.3333, -221.7857) -> (101.3333, -221.7857)
  line L637 (101.3333, -221.7857) -> (101.3333, -215.7857)
  line L638 (101.3333, -215.7857) -> (107.3333, -215.7857)
  line L639 (107.3333, -215.7857) -> (107.3333, -221.7857)
  line L640 (53.6667, -229.6429) -> (47.6667, -229.6429)
  line L641 (47.6667, -229.6429) -> (47.6667, -223.6429)
  line L642 (47.6667, -223.6429) -> (53.6667, -223.6429)
  line L643 (53.6667, -223.6429) -> (53.6667, -229.6429)
  line L644 (61.3333, -229.6429) -> (55.3333, -229.6429)
  line L645 (55.3333, -229.6429) -> (55.3333, -223.6429)
  line L646 (55.3333, -223.6429) -> (61.3333, -223.6429)
  line L647 (61.3333, -223.6429) -> (61.3333, -229.6429)
  line L648 (69, -229.6429) -> (63, -229.6429)
  line L649 (63, -229.6429) -> (63, -223.6429)
  line L650 (63, -223.6429) -> (69, -223.6429)
  line L651 (69, -223.6429) -> (69, -229.6429)
  line L652 (76.6667, -229.6429) -> (70.6667, -229.6429)
  line L653 (70.6667, -229.6429) -> (70.6667, -223.6429)
  line L654 (70.6667, -223.6429) -> (76.6667, -223.6429)
  line L655 (76.6667, -223.6429) -> (76.6667, -229.6429)
  line L656 (84.3333, -229.6429) -> (78.3333, -229.6429)
  line L657 (78.3333, -229.6429) -> (78.3333, -223.6429)
  line L658 (78.3333, -223.6429) -> (84.3333, -223.6429)
  line L659 (84.3333, -223.6429) -> (84.3333, -229.6429)
  line L660 (92, -229.6429) -> (86, -229.6429)
  line L661 (86, -229.6429) -> (86, -223.6429)
  line L662 (86, -223.6429) -> (92, -223.6429)
  line L663 (92, -223.6429) -> (92, -229.6429)
  line L664 (99.6667, -229.6429) -> (93.6667, -229.6429)
  line L665 (93.6667, -229.6429) -> (93.6667, -223.6429)
  line L666 (93.6667, -223.6429) -> (99.6667, -223.6429)
  line L667 (99.6667, -223.6429) -> (99.6667, -229.6429)
  line L668 (107.3333, -229.6429) -> (101.3333, -229.6429)
  line L669 (101.3333, -229.6429) -> (101.3333, -223.6429)
  line L670 (101.3333, -223.6429) -> (107.3333, -223.6429)
  line L671 (107.3333, -223.6429) -> (107.3333, -229.6429)
  line L672 (53.6667, -237.5) -> (47.6667, -237.5)
  line L673 (47.6667, -237.5) -> (47.6667, -231.5)
  line L674 (47.6667, -231.5) -> (53.6667, -231.5)
  line L675 (53.6667, -231.5) -> (53.6667, -237.5)
  line L676 (61.3333, -237.5) -> (55.3333, -237.5)
  line L677 (55.3333, -237.5) -> (55.3333, -231.5)
  line L678 (55.3333, -231.5) -> (61.3333, -231.5)
  line L679 (61.3333, -231.5) -> (61.3333, -237.5)
  line L680 (69, -237.5) -> (63, -237.5)
  line L681 (63, -237.5) -> (63, -231.5)
  line L682 (63, -231.5) -> (69, -231.5)
  line L683 (69, -231.5) -> (69, -237.5)
  line L684 (76.6667, -237.5) -> (70.6667, -237.5)
  line L685 (70.6667, -237.5) -> (70.6667, -231.5)
  line L686 (70.6667, -231.5) -> (76.6667, -231.5)
  line L687 (76.6667, -231.5) -> (76.6667, -237.5)
  line L688 (84.3333, -237.5) -> (78.3333, -237.5)
  line L689 (78.3333, -237.5) -> (78.3333, -231.5)
  line L690 (78.3333, -231.5) -> (84.3333, -231.5)
  line L691 (84.3333, -231.5) -> (84.3333, -237.5)
  line L692 (92, -237.5) -> (86, -237.5)
  line L693 (86, -237.5) -> (86, -231.5)
  line L694 (86, -231.5) -> (92, -231.5)
  line L695 (92, -231.5) -> (92, -237.5)
  line L696 (99.6667, -237.5) -> (93.6667, -237.5)
  line L697 (93.6667, -237.5) -> (93.6667, -231.5)
  line L698 (93.6667, -231.5) -> (99.6667, -231.5)
  line L699 (99.6667, -231.5) -> (99.6667, -237.5)
  line L700 (101.3333, -231.5) -> (107.3333, -231.5)
  line L701 (107.3333, -231.5) -> (107.3333, -237.5)
  line L702 (107.3333, -237.5) -> (101.3333, -237.5)
  line L703 (101.3333, -237.5) -> (101.3333, -231.5)
  line L704 (156, -177) -> (156, -160)
  line L705 (156, -160) -> (143.1111, -160)
  line L706 (143.1111, -160) -> (143.1111, -155)
  line L707 (143.1111, -155) -> (125.2222, -155)
  line L708 (125.2222, -155) -> (125.2222, -160)
  line L709 (125.2222, -160) -> (107.3333, -160)
  line L710 (107.3333, -160) -> (107.3333, -155)
  line L711 (107.3333, -155) -> (89.4444, -155)
  line L712 (89.4444, -155) -> (89.4444, -160)
  line L713 (89.4444, -160) -> (71.5556, -160)
  line L714 (71.5556, -160) -> (71.5556, -155)
  line L715 (71.5556, -155) -> (53.6667, -155)
  line L716 (53.6667, -155) -> (53.6667, -160)
  line L717 (53.6667, -160) -> (35.7778, -160)
  line L718 (35.7778, -160) -> (35.7778, -155)
  line L719 (35.7778, -155) -> (17.8889, -155)
  line L720 (17.8889, -155) -> (17.8889, -160)
  line L721 (17.8889, -160) -> (5, -160)
  line L722 (5, -160) -> (5, -177)
  line L723 (5, -177) -> (0, -177)
  line L724 (0, -177) -> (0, -199)
  line L725 (0, -199) -> (5, -199)
  line L726 (5, -199) -> (5, -221)
  line L727 (5, -221) -> (0, -221)
  line L728 (0, -221) -> (0, -243)
  line L729 (0, -243) -> (5, -243)
  line L730 (5, -243) -> (5, -265)
  line L731 (5, -265) -> (156, -265)
  line L732 (156, -265) -> (156, -243)
  line L733 (156, -243) -> (161, -243)
  line L734 (161, -243) -> (161, -221)
  line L735 (161, -221) -> (156, -221)
  line L736 (156, -221) -> (156, -199)
  line L737 (156, -199) -> (161, -199)
  line L738 (161, -199) -> (161, -177)
  line L739 (161, -177) -> (156, -177)
  circle A0 centre (-78.3333, -37.5) radius 7.5
  circle A1 centre (-78.3333, -62.5) radius 7.5
  circle A2 centre (-78.3333, -87.5) radius 7.5
  circle A3 centre (-78.3333, -112.5) radius 7.5
  line L740 (-93, -5) -> (-93, 0)
  line L741 (-93, 0) -> (-115, 0)
  line L742 (-115, 0) -> (-115, -150)
  line L743 (-115, -150) -> (-93, -150)
  line L744 (-93, -150) -> (-93, -145)
  line L745 (-93, -145) -> (-71, -145)
  line L746 (-71, -145) -> (-71, -150)
  line L747 (-71, -150) -> (-49, -150)
  line L748 (-49, -150) -> (-49, -145)
  line L749 (-49, -145) -> (-27, -145)
  line L750 (-27, -145) -> (-27, -150)
  line L751 (-27, -150) -> (-10, -150)
  line L752 (-10, -150) -> (-10, -136.3636)
  line L753 (-10, -136.3636) -> (-5, -136.3636)
  line L754 (-5, -136.3636) -> (-5, -122.7273)
  line L755 (-5, -122.7273) -> (-10, -122.7273)
  line L756 (-10, -122.7273) -> (-10, -109.0909)
  line L757 (-10, -109.0909) -> (-5, -109.0909)
  line L758 (-5, -109.0909) -> (-5, -95.4545)
  line L759 (-5, -95.4545) -> (-10, -95.4545)
  line L760 (-10, -95.4545) -> (-10, -81.8182)
  line L761 (-10, -81.8182) -> (-5, -81.8182)
  line L762 (-5, -81.8182) -> (-5, -68.1818)
  line L763 (-5, -68.1818) -> (-10, -68.1818)
  line L764 (-10, -68.1818) -> (-10, -54.5455)
  line L765 (-10, -54.5455) -> (-5, -54.5455)
  line L766 (-5, -54.5455) -> (-5, -40.9091)
  line L767 (-5, -40.9091) -> (-10, -40.9091)
  line L768 (-10, -40.9091) -> (-10, -27.2727)
  line L769 (-10, -27.2727) -> (-5, -27.2727)
  line L770 (-5, -27.2727) -> (-5, -13.6364)
  line L771 (-5, -13.6364) -> (-10, -13.6364)
  line L772 (-10, -13.6364) -> (-10, 0)
  line L773 (-10, 0) -> (-27, 0)
  line L774 (-27, 0) -> (-27, -5)
  line L775 (-27, -5) -> (-49, -5)
  line L776 (-49, -5) -> (-49, 0)
  line L777 (-49, 0) -> (-71, 0)
  line L778 (-71, 0) -> (-71, -5)
  line L779 (-71, -5) -> (-93, -5)
component "right panel" placed x (1, 0, 0) y (0, 1, 0) z (0, 0, 1) at (0, 0, 0)
component "front panel" placed x (0, 0, 1) y (-1, 0, 0) z (0, -1, 0) at (150, 0, -150)
component "bottom panel" placed x (0, 0, 1) y (0, 1, 0) z (-1, 0, 0) at (150, 0, -150)
component "back panel" placed x (0, 0, 1) y (1, 0, 0) z (0, 1, 0) at (-11, 161, -150)
component "left panel" placed x (-1, 0, 0) y (0, 1, 0) z (0, 0, -1) at (150, 0, -150)
equation "thickness = 5 mm"
equation "box_length = 150 mm"
equation "box_width = 161 mm"
equation "box_height = 110 mm"
equation "port_radius = 15 mm"
equation "top_button_radius = 15 mm"
equation "top_disk_radius = 50 mm"
equation "little_square = 6 mm"
equation "d9 = box_length"
equation "d10 = box_width"
equation "lfingers = 5"
equation "wfingers = 4"
equation "hfingers = 2"
equation "lfingerw = box_length / ( ( lfingers * 2 ) + 1 )"
equation "wfingerw = box_width / ( ( wfingers * 2 ) + 1 )"
equation "hfingerw = box_height / ( ( hfingers * 2 ) + 1 )"
equation "d17 = thickness"
equation "d19 = lfingerw"
equation "d20 = lfingerw"
equation "d21 = -thickness"
equation "d23 = lfingers"
equation "d25 = -( box_length - ( lfingerw * 3 ) )"
equation "d27 = box_height"
equation "d28 = thickness"
equation "d30 = hfingerw"
equation "d31 = hfingerw"
equation "d32 = -thickness"
equation "d35 = hfingers"
equation "d37 = -( box_height - ( hfingerw * 3 ) )"
equation "d39 = -thickness"
equation "d41 = thickness"
equation "d43 = wfingerw"
equation "d44 = wfingerw"
equation "d45 = -thickness"
equation "d47 = wfingers"
equation "d49 = ( box_width - ( wfingerw * 3 ) )"
equation "d54 = box_width"
equation "d55 = little_square"
equation "d56 = little_square"
equation "d57 = box_width / 3"
equation "num_squares = 8"
equation "d59 = box_length"
equation "dist_between_sqs = 2 mm"
equation "d64 = -( 1 / 3 ) * box_width"
equation "d65 = -1 / 2 * box_height"
equation "d66 = 1 / 4 * box_height"
equation "d68 = -thickness"
equation "d70 = port_radius"
equation "d71 = box_length / 4"
equation "d72 = box_height / 3"
equation "d73 = -thickness"
equation "d77 = -( box_length / 4 * 2 )"
equation "d79 = little_square"
equation "d80 = little_square * 5 / 2"
equation "d81 = box_height / 6"
equation "d82 = box_length / 6"
equation "d83 = -thickness"
equation "d87 = -( box_length / 2 )"
equation "d127 = 55 * 6 mm"
equation "d131 = box_width * 3 / 4"
equation "d132 = box_height / 3"
equation "d134 = box_height / 12"
equation "d135 = box_height / 12"
equation "d136 = box_height / 12"
equation "d137 = box_height / 12"
equation "d138 = box_height / 24"
equation "d139 = box_height / 24"
equation "d145 = ( box_width * 3 / 4 ) - ( ( 2 * 13.801 ) * 1 mm )"
equation "d168 = box_length"
equation "d169 = box_width"
named bodies: "bottom panel", "front panel", "back panel", "left panel", "right panel"
